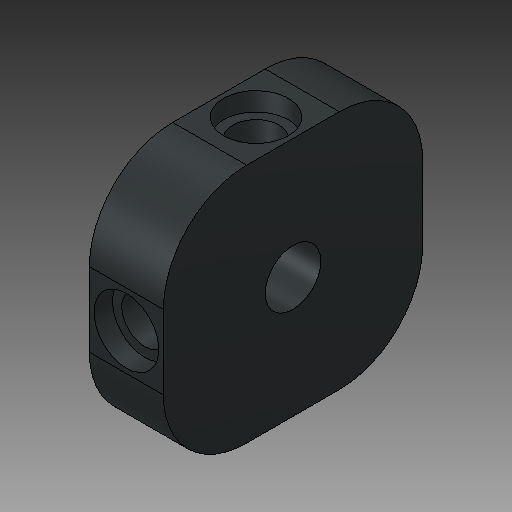
# Autodesk Inventor part: 限位塊
Saved by Autodesk Inventor 2017 (Build 210142000, 142)
## iProperties
Part Number: 限位塊
Material: SS41
Document SubType Name: Modeling
Designer: G
Density: 7.85 g/cm^3
Appearance: 鐵灰色
Author: G
Autodesk Inventor part; units mm, degrees
ref_plane "YZ Plane" through (0, 0, 0) normal (1, 0, 0) x (0, 1, 0)
ref_plane "XZ Plane" through (0, 0, 0) normal (0, 1, 0) x (-1, 0, 0)
ref_plane "XY Plane" through (0, 0, 0) normal (0, 0, 1) x (1, 0, 0)
sketch "草圖4" plane through (0, 0, 0) normal (1, 0, 0) x (0, 1, 0)
  line L0 (4, 14) -> (-4, 14)
  line L1 (-13, 5) -> (-13, -5)
  line L2 (-4, -14) -> (4, -14)
  line L3 (13, -5) -> (13, 5)
  arc A0 (13, 5) -> (4, 14) centre (4, 5) ccw
  arc A1 (4, -14) -> (13, -5) centre (4, -5) ccw
  arc A2 (-13, -5) -> (-4, -14) centre (-4, -5) ccw
  arc A3 (-4, 14) -> (-13, 5) centre (-4, 5) ccw
  circle A4 centre (0, 0) radius 3
  point P0 (-13, -14)
  point P1 (-13, 14)
  point P2 (13, -14)
  point P3 (0, 14)
  point P4 (13, 0)
  dimension "d13" = 26
  dimension "d14" = 28
  dimension "d15" = 9
  dimension "d23" = 6
  constraints: 8 end point, 8 point on circle, 8 tangent, 6 point on line, 5 centre point, 3 equal radius, 2 midpoint, 2 parallel, 1 coincident, 1 horizontal, 1 horizontal alignment, 1 perpendicular, 1 vertical alignment
  measures "d13" distance of point (13, -14) point (-13, -14)
  measures "d14" distance of point (-13, -14) point (-13, 14)
  measures "d15" radius of A0
  measures "d23" diameter of A4
extrude "擠出1" add sketch "草圖4" along normal mid plane 8
sketch "草圖3" plane through (0, 0, 0) normal (0, 0, 1) x (1, 0, 0)
  line L0 (0, 13) -> (3.5, 13)
  line L1 (3.5, 13) -> (3.5, 11)
  line L2 (3.5, 11) -> (2.5, 11)
  line L3 (2.5, 11) -> (2.5, 7)
  line L4 (2.5, 7) -> (0, 7)
  line L5 (0, 13) -> (0, 7)
  line L6 (4, 13) -> (-4, 13) construction
  point P0 (0, 0)
  dimension "d5" = 2
  dimension "d6" = 7
  dimension "d7" = 6
  dimension "d8" = 5
  constraints: 12 end point, 2 vertical, 1 horizontal, 1 midpoint, 1 parallel, 1 perpendicular, 1 point on line
  measures "d5" distance of L0.end L1.end
  measures "d6" diameter of L1 L5
  measures "d7" distance between parallel lines of L4 L0
  measures "d8" diameter of L3 L5
revolve "迴轉2" cut sketch "草圖3" angle 360 about axis through (0, 13, 0) along (0, -1, 0)
sketch "草圖5" plane through (0, 0, 0) normal (1, 0, 0) x (0, 1, 0)
  line L0 (0, 14) -> (3.5, 14)
  line L1 (3.5, 14) -> (3.5, 12)
  line L2 (3.5, 12) -> (2.5, 12)
  line L3 (2.5, 12) -> (2.5, 8)
  line L4 (2.5, 8) -> (0, 8)
  line L5 (0, 14) -> (0, 8)
  line L6 (-4, 14) -> (4, 14) construction
  point P0 (0, 0)
  point P1 (0, 0)
  dimension "d18" = 2
  dimension "d19" = 7
  dimension "d20" = 6
  dimension "d21" = 5
  constraints: 12 end point, 2 vertical, 1 horizontal, 1 midpoint, 1 parallel, 1 perpendicular, 1 point on line
  measures "d18" distance of L0.end L1.end
  measures "d19" diameter of L1 L5
  measures "d20" distance between parallel lines of L4 L0
  measures "d21" diameter of L3 L5
revolve "迴轉3" cut sketch "草圖5" angle 360 about axis through (0, 0, 14) along (0, 0, -1)
pattern_circular "環形陣列1" count 2 over 360 about axis through (-10, 0, 0) along (1, 0, 0) of "迴轉2", "迴轉3"
